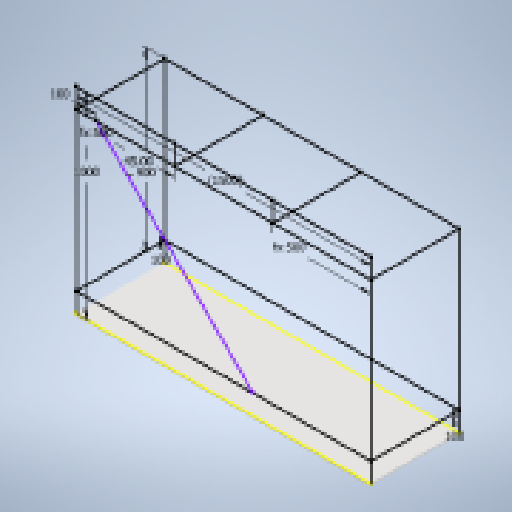
# Autodesk Inventor part: roller conveyor 1
Saved by Autodesk Inventor 2023.1 (Build 271208000, 208)
## iProperties
Created: 2023-08-25
Part Number: roller conveyor 1
Material: Generic
Document SubType Name: Modeling
Designer: admin
Density: 1 g/cm^3
Appearance: Default
Author: admin
Autodesk Inventor part; units mm, degrees
ref_plane "YZ Plane" through (0, 0, 0) normal (1, 0, 0) x (0, 1, 0)
ref_plane "XZ Plane" through (0, 0, 0) normal (0, 1, 0) x (-1, 0, 0)
ref_plane "XY Plane" through (0, 0, 0) normal (0, 0, 1) x (1, 0, 0)
sketch "Sketch1" plane through (0, 0, 0) normal (0, 1, 0) x (-1, 0, 0)
  line L0 (750, -225) -> (-750, -225)
  line L1 (-750, -225) -> (-750, 225)
  line L2 (-750, 225) -> (750, 225)
  line L3 (750, 225) -> (750, -225)
  line L4 (750, -225) -> (-750, 225) construction
  line L5 (-750, -225) -> (750, 225) construction
  point P0 (0, 0)
  dimension "d0" = 1500
  dimension "d1" = 450
  constraints: 12 end point, 2 midpoint, 2 parallel, 1 horizontal, 1 perpendicular
  measures "d0" distance of L1.end L2.end
  measures "d1" distance of L0.end L1.end
extrude "Extrusion1" add sketch "Sketch1" against normal blind 10
sketch3d "3D Sketch1"
equation "\"d10\" = 0.333333 * d9"
equation "\"d11\" = d10"
equation "\"d16\" = d10"
equation "\"d17\" = d10"
equation "\"d9\" = 1500"
body "Solid1"
